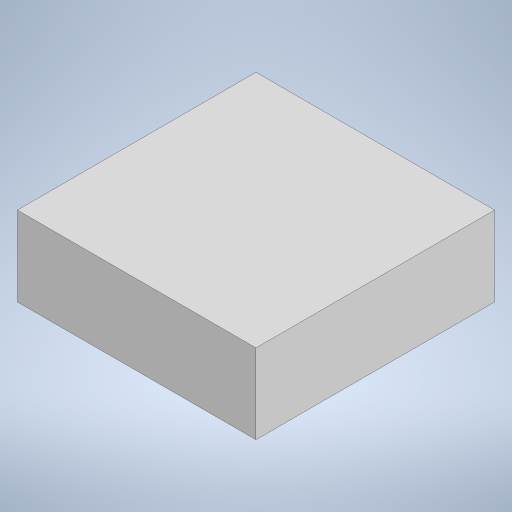
# Autodesk Inventor part: keypad cover
Saved by Autodesk Inventor 2023 (Build 270158000, 158)
## iProperties
Created: 2022-12-19
Part Number: keypad cover
Material: Generic
Document SubType Name: Modeling
Designer: appab
Density: 1 g/cm^3
Appearance: Default
Author: appab
Autodesk Inventor part; units mm, degrees
ref_plane "YZ Plane" through (0, 0, 0) normal (1, 0, 0) x (0, 1, 0)
ref_plane "XZ Plane" through (0, 0, 0) normal (0, 1, 0) x (-1, 0, 0)
ref_plane "XY Plane" through (0, 0, 0) normal (0, 0, 1) x (1, 0, 0)
sketch "Sketch1" plane through (0, 0, 0) normal (0, 1, 0) x (-1, 0, 0)
  line L0 (-70.485, -70.485) -> (5.715, -70.485)
  line L1 (5.715, -70.485) -> (5.715, 5.715)
  line L2 (5.715, 5.715) -> (-70.485, 5.715)
  line L3 (-70.485, 5.715) -> (-70.485, -70.485)
  line L4 (-70.485, -70.485) -> (5.715, 5.715) construction
  line L5 (5.715, -70.485) -> (-70.485, 5.715) construction
  line L6 (5.715, 5.715) -> (0.635, 5.715) construction
  line L7 (0.635, 5.715) -> (0.635, 0.635) construction
  line L8 (0.635, 0.635) -> (5.715, 0.635) construction
  line L9 (5.715, 0.635) -> (5.715, 5.715) construction
  line L10 (-3.175, -3.175) -> (-61.595, -3.175)
  line L11 (-61.595, -3.175) -> (-61.595, -61.595)
  line L12 (-61.595, -61.595) -> (-3.175, -61.595)
  line L13 (-3.175, -61.595) -> (-3.175, -3.175)
  line L14 (-3.175, -3.175) -> (-61.595, -61.595) construction
  line L15 (-61.595, -3.175) -> (-3.175, -61.595) construction
  circle A0 centre (0.635, 0.635) radius 1.7399
  circle A1 centre (0.635, -65.405) radius 1.7399
  circle A2 centre (-65.405, 0.635) radius 1.7399
  circle A3 centre (-65.405, -65.405) radius 1.7399
  point P0 (0, 0)
  point P1 (-32.385, -32.385)
  dimension "d2" = 76.2
  dimension "d3" = 76.2
  dimension "d4" = 5.08
  dimension "d5" = 5.08
  dimension "d7" = 58.42
  dimension "d8" = 58.42
  dimension "d9" = 3.4798
  dimension "d12" = 66.04
  dimension "d15" = 66.04
  constraints: 32 end point, 6 parallel, 4 centre point, 4 horizontal, 4 midpoint, 3 perpendicular, 1 coincident, 1 vertical, 6 other
  measures "d2" distance of L2.end L1.end
  measures "d3" distance of L1.end L0.end
  measures "d4" distance of L8.end L7.end
  measures "d5" distance of L7.end L6.end
  measures "d7" distance of L12.end L11.end
  measures "d8" distance of L11.end L10.end
  measures "d9" diameter of A0
  measures "d12" distance of A0.centre A1.centre
  measures "d15" distance of A0.centre A2.centre
extrude "Extrusion1" add sketch "Sketch1" along normal blind 22.86
sketch "Sketch2" plane through (0, 22.86, 0) normal (0, 1, 0) x (1, 0, 0)
  line L0 (-5.715, -5.715) -> (70.485, -5.715) projected
  line L1 (70.485, -5.715) -> (70.485, 70.485) projected
  line L2 (-5.715, -5.715) -> (70.485, -5.715)
  line L3 (70.485, -5.715) -> (70.485, 70.485)
  line L4 (70.485, 70.485) -> (-5.715, 70.485)
  line L5 (-5.715, 70.485) -> (-5.715, -5.715)
  point P0 (0, 0)
  constraints: 8 end point, 2 parallel, 1 horizontal, 1 perpendicular
extrude "Extrusion2" add sketch "Sketch2" along normal blind 2.54
sketch "Sketch3" plane through (-5.715, 0, -70.485) normal (-1, 0, 0) x (0, 0, 1)
  line L0 (38.1, 0) -> (38.1, 25.4) construction
  line L1 (76.2, 25.4) -> (0, 25.4) construction
  line L2 (38.1, 0) -> (40.005, 0) construction
  line L3 (40.005, 0) -> (36.195, 0)
  line L4 (36.195, 0) -> (36.195, 1.27)
  line L5 (40.005, 1.27) -> (40.005, 0)
  arc A0 (40.005, 1.27) -> (36.195, 1.27) centre (38.1, 1.27) ccw
  point P0 (70.485, 0)
  point P1 (38.1, 3.175)
  dimension "d24" = 1.27
  dimension "d25" = 3.81
  dimension "d26" = 1.905
  constraints: 10 end point, 3 point on circle, 1 centre point, 1 horizontal, 1 midpoint, 1 parallel, 1 perpendicular, 1 point on line
  measures "d24" distance of L3.end L4.end
  measures "d25" distance of L2.end L3.end
  measures "d26" distance of point (38.1, 3.175) A0.centre
extrude "Extrusion3" cut sketch "Sketch3" against normal up to surface (8.89 mm away)
sketch "Sketch4" plane through (0, 0, 0) normal (0, -1, 0) x (1, 0, 0)
  line L0 (61.595, -3.175) -> (3.175, -3.175) construction
  line L1 (-5.715, 5.715) -> (70.485, 5.715) construction
  line L2 (3.175, -3.175) -> (61.595, -3.175)
  line L3 (61.595, -3.175) -> (61.595, 1.27)
  line L4 (61.595, 1.27) -> (3.175, 1.27)
  line L5 (3.175, 1.27) -> (3.175, -3.175)
  line L6 (70.485, -70.485) -> (-5.715, -70.485) construction
  circle A0 centre (32.385, -32.385) radius 4.575 construction
  line L7 (-1.27, -61.595) -> (3.175, -61.595)
  line L8 (3.175, -61.595) -> (3.175, -3.175)
  line L9 (3.175, -3.175) -> (-1.27, -3.175)
  line L10 (-1.27, -3.175) -> (-1.27, -61.595)
  line L11 (61.595, -66.04) -> (61.595, -61.595)
  line L12 (61.595, -61.595) -> (3.175, -61.595)
  line L13 (3.175, -61.595) -> (3.175, -66.04)
  line L14 (3.175, -66.04) -> (61.595, -66.04)
  line L15 (66.04, -3.175) -> (61.595, -3.175)
  line L16 (61.595, -3.175) -> (61.595, -61.595)
  line L17 (61.595, -61.595) -> (66.04, -61.595)
  line L18 (66.04, -61.595) -> (66.04, -3.175)
  point P0 (0, 0)
  dimension "d31" = 360
  constraints: 32 end point, 2 parallel, 1 centre point, 1 horizontal, 1 perpendicular, 33 other
extrude "Extrusion4" cut sketch "Sketch4" against normal blind 22.86 contours L5 L4 L3 L2 | L8 L7 L10 L9 | L15 L18 L17 L16 | L12 L11 L14 L13
body "Solid1"
